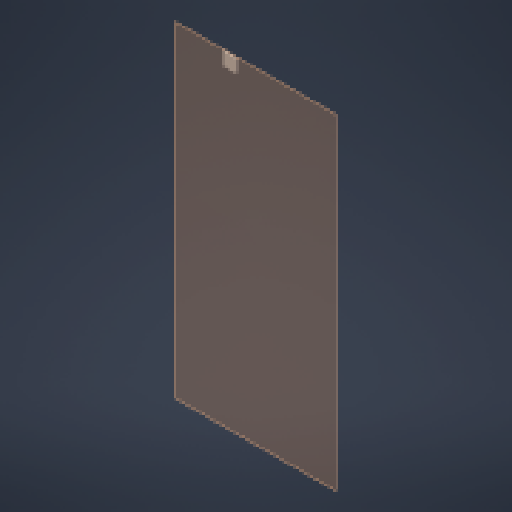
# Autodesk Inventor part: 0001
Saved by Autodesk Inventor 2024 (Build 280153000, 153)
## iProperties
Created: 2023-05-19
Part Number: 0001
Material: Genérico
Document SubType Name: Sheet Metal
Designer: javie
Density: 1 g/cm^3
Sheet Metal Rule: Por defecto_mm
Appearance: Valor por defecto
Author: javie
Autodesk Inventor part; units mm, degrees
ref_plane "YZ Plane" through (0, 0, 0) normal (1, 0, 0) x (0, 1, 0)
ref_plane "XZ Plane" through (0, 0, 0) normal (0, 1, 0) x (-1, 0, 0)
ref_plane "XY Plane" through (0, 0, 0) normal (0, 0, 1) x (1, 0, 0)
ref_plane "Plano de trabajo1" through (0, 0, 0) normal (0, 0, 1) x (1, 0, 0)
sketch "Boceto1" plane through (0, 0, 0) normal (0, 0, 1) x (1, 0, 0)
  line L0 (-164.2, 333) -> (-44.2, 333)
  line L1 (-44.2, 333) -> (-44.2, 363)
  line L2 (-44.2, 363) -> (-164.2, 363)
  line L3 (-164.2, 363) -> (-164.2, 333)
  line L4 (-134.2, 363) -> (-104.2, 363)
  line L5 (-104.2, 363) -> (-104.2, 333)
  line L6 (-104.2, 333) -> (-134.2, 333)
  line L7 (-134.2, 333) -> (-134.2, 363)
  line L8 (-74.2, 363) -> (-74.2, 333)
  point P0 (0, 0)
  point P1 (-44.2, 348)
  point P2 (-134.2, 348)
  dimension "d0" = 120
  dimension "d1" = 30
  dimension "d2" = 30
  dimension "d3" = 30
  dimension "d4" = 30
  constraints: 18 end point, 4 parallel, 3 midpoint, 3 perpendicular, 3 point on line, 2 horizontal
  measures "d0" distance of L2.end L1.end
  measures "d1" distance of L1.end L0.end
  measures "d2" distance of L5.end L6.end
  measures "d3" distance from line of point (-44.2, 348) L8
  measures "d4" distance from line of L3 point (-134.2, 348)
extrude "Extrusión1" add sketch "Boceto1" against normal blind 2 contours L8 L2 L1 L0
equation "\"Radio_pliegue\" = Grosor"
equation "\"Anchura_desahogo_plegado\" = Grosor"
equation "\"Profundidad_desahogo_plegado\" = 0.5 * Grosor"
equation "\"Tamaño_destalonado\" = 4 * Grosor"
equation "\"Remanente_mínimo\" = 2 * Grosor"
equation "\"Radiodetransición\" = Radio_pliegue"
equation "\"Tamaño_de_radio_de_Jacobi\" = Radio_pliegue"
equation "\"TamañoSeparación\" = Grosor"
equation "\"Grosor\" = 0.5"
